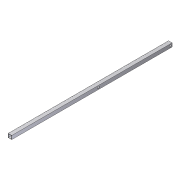
# Autodesk Inventor part: FE-00002-05
Saved by Autodesk Inventor 2012 (Build 160160000, 160)
## iProperties
Created: 2008-05-14
Part Number: FE-00002-05
Document SubType Name: Modeling
Designer: narosenberg
Density: 1 g/cm^3
Mass: 1028.66 g
Surface Area: 6502.61 cm^2
Volume: 1028.66 cm^3
Material: Default
Author: narosenberg
Autodesk Inventor part; units mm, degrees
ref_plane "YZ Plane" through (0, 0, 0) normal (1, 0, 0) x (0, 1, 0)
ref_plane "XZ Plane" through (0, 0, 0) normal (0, 1, 0) x (-1, 0, 0)
ref_plane "XY Plane" through (0, 0, 0) normal (0, 0, 1) x (1, 0, 0)
sketch "Sketch1" plane through (0, 0, 0) normal (0, 0, 1) x (1, 0, 0)
  line L0 (-31.3178, 22.4806) -> (13.1322, 22.4806)
  line L1 (13.1322, 22.4806) -> (13.1322, -21.9694)
  line L2 (13.1322, -21.9694) -> (-31.3178, -21.9694)
  line L3 (-31.3178, -21.9694) -> (-31.3178, 22.4806)
  dimension "d0" = 44.45
  dimension "d1" = 44.45
  constraints: 8 end point, 2 parallel, 1 horizontal, 1 perpendicular
  measures "d0" distance of L0.start L0.end
  measures "d1" distance of L0.end L1.end
extrude "Extrusion1" add sketch "Sketch1" along normal blind 1981.2
shell "Shell1" thickness 3.175 removed faces 2 at (-16.5012, 7.664, 0) at (-16.5012, 7.664, 1981.2)
sketch "Sketch2" plane through (13.1322, -21.9694, 0) normal (1, 0, 0) x (0, 0, -1)
  line L0 (0, 44.45) -> (0, 0) projected
  line L1 (0, 44.45) -> (-1981.2, 44.45) projected
  circle A0 centre (-911.225, 22.225) radius 18.2563
  circle A1 centre (-22.225, 22.225) radius 18.2563
  dimension "d5" = 36.5125
  dimension "d6" = 44.45
  dimension "d7" = 22.225
  dimension "d16" = 36.5125
  dimension "d17" = 22.225
  dimension "d18" = 889
  constraints: 2 centre point, 1 horizontal alignment
  measures "d5" diameter of A0
  measures "d6" distance of L0.start L0.end
  measures "d7" distance from line of L1 A0.centre
  measures "d16" diameter of A1
  measures "d17" distance from line of A1.centre L0
  measures "d18" distance of A0.centre A1.centre
extrude "Extrusion2" cut sketch "Sketch2" against normal through all
sketch "Sketch4" plane through (13.1322, -21.9694, 0) normal (1, 0, 0) x (0, 0, -1)
  circle A0 centre (-911.225, 22.225) radius 18.2562 projected
  circle A1 centre (-911.225, 22.225) radius 12.7
  circle A2 centre (-22.225, 22.225) radius 18.2562 projected
  circle A3 centre (-22.225, 22.225) radius 12.7
  dimension "d20" = 25.4
  dimension "d23" = 25.4
  constraints: 2 centre point, 2 coincident
  measures "d20" diameter of A1
  measures "d23" diameter of A3
extrude "Extrusion4" add sketch "Sketch4" against normal blind 3.175
equation "\"d1\" = d0"
equation "\"d7\" = 0.5 * d6"
equation "\"d16\" = d5"
body "Solid1"
